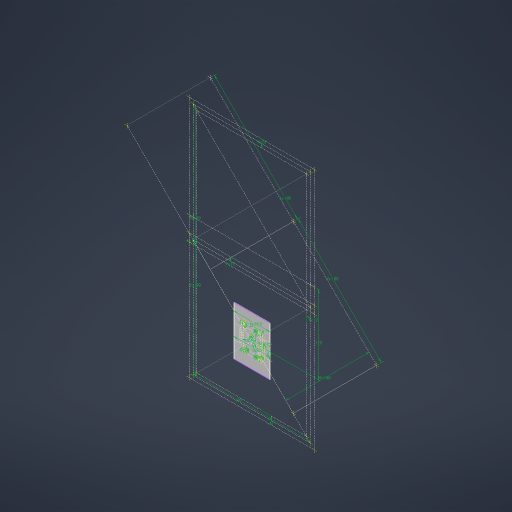
# Autodesk Inventor part: chassis
Saved by Autodesk Inventor 2023.5 (Build 275446000, 446)
## iProperties
Created: 2025-01-19
Part Number: chassis
Material: 一般
Document SubType Name: Modeling
Designer: IshiiLabHonda
Density: 1 g/cm^3
Appearance: 既定
Author: IshiiLabHonda
Autodesk Inventor part; units mm, degrees
ref_plane "YZ Plane" through (0, 0, 0) normal (1, 0, 0) x (0, 1, 0)
ref_plane "XZ Plane" through (0, 0, 0) normal (0, 1, 0) x (-1, 0, 0)
ref_plane "XY Plane" through (0, 0, 0) normal (0, 0, 1) x (1, 0, 0)
sketch "スケッチ1" plane through (0, 0, 0) normal (0, 0, 1) x (1, 0, 0)
  line L0 (-90, 90) -> (90, 90) construction
  line L1 (90, 90) -> (90, -90) construction
  line L2 (90, -90) -> (-90, -90) construction
  line L3 (-90, -90) -> (-90, 90) construction
  line L4 (-90, 90) -> (-90, 270) construction
  line L5 (-90, 270) -> (90, 270) construction
  line L6 (90, 270) -> (90, 90) construction
  line L7 (-90, 90) -> (90, -90) construction
  line L8 (90, 90) -> (-90, -90) construction
  line L9 (0, 0) -> (0, 10) construction
  line L10 (0, 0) -> (10, 0) construction
  line L11 (-90, 270) -> (90, 90) construction
  line L12 (-90, 90) -> (90, 270) construction
  line L13 (-96, 276) -> (96, 276) construction
  line L14 (96, 276) -> (96, -96) construction
  line L15 (96, -96) -> (-96, -96) construction
  line L16 (-96, -96) -> (-96, 276) construction
  line L17 (-84, 264) -> (84, 264) construction
  line L18 (84, 264) -> (84, -84) construction
  line L19 (84, -84) -> (-84, -84) construction
  line L20 (-84, -84) -> (-84, 264) construction
  line L21 (-96, 96) -> (96, 96) construction
  line L22 (-96, 84) -> (96, 84) construction
  line L23 (-63.6396, 63.6396) -> (63.6396, 190.9188) construction
  line L24 (63.6396, 190.9188) -> (190.9188, 63.6396) construction
  line L25 (190.9188, 63.6396) -> (63.6396, -63.6396) construction
  line L26 (63.6396, -63.6396) -> (-63.6396, 63.6396) construction
  line L27 (-190.9188, 190.9188) -> (-63.6396, 318.1981) construction
  line L28 (-63.6396, 318.1981) -> (63.6396, 190.9188) construction
  line L29 (-63.6396, 63.6396) -> (-190.9188, 190.9188) construction
  line L30 (-96, 120) -> (96, 120) construction
  point P0 (-63.6396, 318.1981)
  point P1 (-90, 120)
  point P2 (90, 120)
  dimension "d8" = 10
  dimension "d9" = 10
  dimension "d10" = 12
  dimension "d11" = 12
  dimension "d12" = 12
  dimension "d13" = 12
  dimension "d14" = 180
  dimension "d15" = 180
  dimension "d16" = 180
  dimension "d17" = 12
  dimension "d34" = 180
  dimension "d35" = 180
  dimension "d36" = 180
  dimension "d37" = 120
  constraints: 62 end point, 13 parallel, 10 point on line, 9 perpendicular, 3 coincident, 2 midpoint, 1 horizontal, 6 other
  measures "d8" distance of L9.start L9.end
  measures "d9" distance of L9.start L10.end
  measures "d10" distance between parallel lines of L15 L19
  measures "d11" distance between parallel lines of L16 L20
  measures "d12" distance between parallel lines of L14 L18
  measures "d13" distance between parallel lines of L17 L13
  measures "d14" distance of L1.end L2.end
  measures "d15" distance of L2.end L0.start
  measures "d16" distance between parallel lines of L0 L5
  measures "d17" distance between parallel lines of L22 L21
  measures "d34" distance between parallel lines of L26 L24
  measures "d35" distance of L23.end L24.end
  measures "d36" distance between parallel lines of L23 L27
  measures "d37" distance between parallel lines of L10 L30
sketch "スケッチ2" plane through (0, 0, 0) normal (0, 0, 1) x (1, 0, 0)
  line L0 (63.6396, 190.9188) -> (190.9188, 63.6396) construction
  line L1 (-63.6396, 318.1981) -> (63.6396, 190.9188) construction
  line L2 (-84, 264) -> (84, 264) construction
  line L3 (-90, 270) -> (90, 270) construction
  line L4 (90, 270) -> (90, 90) construction
  line L5 (-96, 276) -> (96, 276) construction
  line L6 (-90, 90) -> (90, 270) construction
  line L7 (-90, 270) -> (90, 90) construction
  line L8 (-63.6396, 63.6396) -> (63.6396, 190.9188) construction
  line L9 (-96, 120) -> (96, 120) construction
  line L10 (-90, 90) -> (90, 90) construction
  line L11 (-96, 96) -> (96, 96) construction
  line L12 (-96, 84) -> (96, 84) construction
  line L13 (90, -90) -> (-90, -90) construction
  line L14 (0, 0) -> (0, 10) construction
  line L15 (0, 0) -> (10, 0) construction
  line L16 (190.9188, 63.6396) -> (63.6396, -63.6396) construction
  line L17 (63.6396, -63.6396) -> (-63.6396, 63.6396) construction
  line L18 (84, -84) -> (-84, -84) construction
  line L19 (96, -96) -> (-96, -96) construction
  line L20 (-90, 90) -> (-90, 270) construction
  line L21 (-63.6396, 63.6396) -> (-190.9188, 190.9188) construction
  line L22 (-190.9188, 190.9188) -> (-63.6396, 318.1981) construction
  line L23 (96, 276) -> (96, -96) construction
  line L24 (-96, -96) -> (-96, 276) construction
  line L25 (84, 264) -> (84, -84) construction
  line L26 (-84, -84) -> (-84, 264) construction
  line L27 (90, 90) -> (90, -90) construction
  line L28 (-90, 90) -> (90, -90) construction
  line L29 (90, 90) -> (-90, -90) construction
  line L30 (-90, -90) -> (-90, 90) construction
  circle A0 centre (0, 0) radius 15 construction
  circle A1 centre (0, 0) radius 7.5 construction
  line L31 (19, 11.5) -> (27.75, 11.5) construction
  line L32 (27.75, 11.5) -> (27.75, -11.5) construction
  line L33 (27.75, -11.5) -> (19, -11.5) construction
  line L34 (19, -11.5) -> (19, 11.5) construction
  line L35 (19, 11.5) -> (17, 11.5) construction
  line L36 (17, 11.5) -> (17, -11.5) construction
  line L37 (17, -11.5) -> (19, -11.5) construction
  line L38 (17, 1.5) -> (16, 1.5) construction
  line L39 (16, -1.5) -> (17, -1.5) construction
  line L40 (-16, 20) -> (16, 20) construction
  line L41 (16, 20) -> (16, -20) construction
  line L42 (16, -20) -> (-16, -20) construction
  line L43 (-16, -20) -> (-16, 20) construction
  line L44 (-19, 11.5) -> (-27.75, 11.5) construction
  line L45 (-27.75, 11.5) -> (-27.75, -11.5) construction
  line L46 (-27.75, -11.5) -> (-19, -11.5) construction
  line L47 (-19, -11.5) -> (-19, 11.5) construction
  line L48 (-19, 11.5) -> (-17, 11.5) construction
  line L49 (-17, 11.5) -> (-17, -11.5) construction
  line L50 (-17, -11.5) -> (-19, -11.5) construction
  line L51 (-17, 1.5) -> (-16, 1.5) construction
  line L52 (-16, -1.5) -> (-17, -1.5) construction
  line L53 (-13.5, 20) -> (-13.5, -20) construction
  line L54 (13.5, 20) -> (13.5, -20) construction
  line L55 (-9.5, 20) -> (-9.5, 15) construction
  line L56 (-9.5, 15) -> (-13.5, 15) construction
  line L57 (-13.5, 20) -> (-9.5, 15) construction
  line L58 (-9.5, 20) -> (-13.5, 15) construction
  circle A2 centre (-11.5, 17.5) radius 0.8 construction
  line L59 (9.5, 20) -> (9.5, 15) construction
  line L60 (9.5, 15) -> (13.5, 15) construction
  line L61 (9.5, 20) -> (13.5, 15) construction
  line L62 (9.5, 15) -> (13.5, 20) construction
  circle A3 centre (11.5, 17.5) radius 0.8 construction
  line L63 (-13.5, -15) -> (-9.5, -15) construction
  line L64 (-9.5, -15) -> (-9.5, -20) construction
  line L65 (9.5, -20) -> (9.5, -15) construction
  line L66 (9.5, -15) -> (13.5, -15) construction
  line L67 (-13.5, -15) -> (-9.5, -20) construction
  line L68 (-9.5, -15) -> (-13.5, -20) construction
  circle A4 centre (-11.5, -17.5) radius 0.8 construction
  line L69 (9.5, -15) -> (13.5, -20) construction
  line L70 (13.5, -15) -> (9.5, -20) construction
  circle A5 centre (11.5, -17.5) radius 0.8 construction
  point P0 (90, 120)
  point P1 (-90, 120)
  point P2 (-63.6396, 318.1981)
  dimension "d38" = 30
  dimension "d39" = 15
  dimension "d40" = 8.75
  dimension "d41" = 2
  dimension "d42" = 23
  dimension "d44" = 3
  dimension "d45" = 1
  dimension "d46" = 32
  dimension "d48" = 2.5
  dimension "d49" = 20
  dimension "d50" = 20
  dimension "d51" = 1.6
  dimension "d52" = 5
  dimension "d53" = 4
  dimension "d54" = 1.6
  dimension "d55" = 4
  dimension "d56" = 5
  dimension "d57" = 1.6
  dimension "d58" = 4
  dimension "d59" = 5
  dimension "d60" = 1.6
  dimension "d61" = 5
  dimension "d62" = 4
  dimension "d63" = 55.5
  constraints: 80 end point, 18 point on line, 12 parallel, 10 symmetric about line, 6 centre point, 6 perpendicular, 4 midpoint, 2 coincident, 2 collinear, 5 other
  measures "d38" diameter of A0
  measures "d39" diameter of A1
  measures "d40" distance between parallel lines of L34 L32
  measures "d41" distance between parallel lines of L36 L34
  measures "d42" distance between parallel lines of L33 L31
  measures "d44" distance between parallel lines of L39 L38
  measures "d45" distance between parallel lines of L41 L36
  measures "d46" distance between parallel lines of L41 L43
  measures "d48" distance between parallel lines of L43 L53
  measures "d49" distance between parallel lines of L42 L15
  measures "d50" distance between parallel lines of L15 L40
  measures "d51" diameter of A2
  measures "d52" distance of L55.start L55.end
  measures "d53" distance of L55.end L56.end
  measures "d54" diameter of A3
  measures "d55" distance of L59.end L60.end
  measures "d56" distance of L59.start L59.end
  measures "d57" diameter of A4
  measures "d58" distance of L63.start L63.end
  measures "d59" distance of L63.end L64.end
  measures "d60" diameter of A5
  measures "d61" distance of L65.start L65.end
  measures "d62" distance of L65.end L66.end
  measures "d63" distance between parallel lines of L32 L45
sketch "スケッチ3" plane through (0, 0, 0) normal (0, 0, 1) x (1, 0, 0)
  line L0 (63.6396, 190.9188) -> (190.9188, 63.6396) construction
  line L1 (-63.6396, 318.1981) -> (63.6396, 190.9188) construction
  line L2 (-84, 264) -> (84, 264) construction
  line L3 (-90, 270) -> (90, 270) construction
  line L4 (90, 270) -> (90, 90) construction
  line L5 (-96, 276) -> (96, 276) construction
  line L6 (-90, 90) -> (90, 270) construction
  line L7 (-90, 270) -> (90, 90) construction
  line L8 (-63.6396, 63.6396) -> (63.6396, 190.9188) construction
  line L9 (-96, 120) -> (96, 120) construction
  line L10 (-90, 90) -> (90, 90) construction
  line L11 (-96, 96) -> (96, 96) construction
  line L12 (-96, 84) -> (96, 84) construction
  line L13 (90, -90) -> (-90, -90) construction
  line L14 (0, 0) -> (0, 10) construction
  line L15 (0, 0) -> (10, 0) construction
  line L16 (190.9188, 63.6396) -> (63.6396, -63.6396) construction
  line L17 (63.6396, -63.6396) -> (-63.6396, 63.6396) construction
  line L18 (84, -84) -> (-84, -84) construction
  line L19 (96, -96) -> (-96, -96) construction
  line L20 (-90, 90) -> (-90, 270) construction
  line L21 (-63.6396, 63.6396) -> (-190.9188, 190.9188) construction
  line L22 (-190.9188, 190.9188) -> (-63.6396, 318.1981) construction
  line L23 (96, 276) -> (96, -96) construction
  line L24 (-96, -96) -> (-96, 276) construction
  line L25 (84, 264) -> (84, -84) construction
  line L26 (-84, -84) -> (-84, 264) construction
  line L27 (90, 90) -> (90, -90) construction
  line L28 (-90, 90) -> (90, -90) construction
  line L29 (90, 90) -> (-90, -90) construction
  line L30 (-90, -90) -> (-90, 90) construction
  line L31 (-17, 1.5) -> (-16, 1.5) construction
  line L32 (-16, -1.5) -> (-17, -1.5) construction
  line L33 (-19, 11.5) -> (-17, 11.5) construction
  line L34 (-27.75, 11.5) -> (-27.75, -11.5) construction
  line L35 (63.6396, -63.6396) -> (-63.6396, 63.6396) construction
  line L36 (84, -84) -> (-84, -84) construction
  line L37 (-90, -90) -> (-90, 90) construction
  line L38 (96, -96) -> (-96, -96) construction
  line L39 (-90, 90) -> (90, 90) construction
  line L40 (90, -90) -> (-90, -90) construction
  line L41 (90, 90) -> (-90, -90) construction
  line L42 (-90, 90) -> (90, -90) construction
  line L43 (90, 90) -> (90, -90) construction
  line L44 (-27.75, -11.5) -> (-19, -11.5) construction
  line L45 (-19, 11.5) -> (-27.75, 11.5) construction
  line L46 (-17, 11.5) -> (-17, -11.5) construction
  line L47 (-17, -11.5) -> (-19, -11.5) construction
  line L48 (0, 0) -> (0, 10) construction
  line L49 (0, 0) -> (10, 0) construction
  circle A0 centre (0, 0) radius 15 construction
  circle A1 centre (0, 0) radius 7.5 construction
  line L50 (-13.5, 20) -> (-13.5, -20) construction
  line L51 (-16, 20) -> (16, 20) construction
  line L52 (-16, -20) -> (-16, 20) construction
  line L53 (16, -20) -> (-16, -20) construction
  line L54 (-13.5, -15) -> (-9.5, -15) construction
  circle A2 centre (-11.5, -17.5) radius 0.8 projected
  line L55 (-9.5, -15) -> (-13.5, -20) construction
  line L56 (-13.5, -15) -> (-9.5, -20) construction
  line L57 (-63.6396, 318.1981) -> (63.6396, 190.9188) construction
  line L58 (-84, 264) -> (84, 264) construction
  line L59 (-90, 270) -> (90, 270) construction
  line L60 (90, 270) -> (90, 90) construction
  line L61 (-96, 276) -> (96, 276) construction
  line L62 (-90, 90) -> (90, 270) construction
  line L63 (-90, 270) -> (90, 90) construction
  line L64 (-63.6396, 63.6396) -> (63.6396, 190.9188) construction
  line L65 (-96, 120) -> (96, 120) construction
  line L66 (-96, 96) -> (96, 96) construction
  line L67 (-96, 84) -> (96, 84) construction
  line L68 (84, 264) -> (84, -84) construction
  line L69 (96, 276) -> (96, -96) construction
  line L70 (-96, -96) -> (-96, 276) construction
  line L71 (-84, -84) -> (-84, 264) construction
  line L72 (-63.6396, 63.6396) -> (-190.9188, 190.9188) construction
  line L73 (-90, 90) -> (-90, 270) construction
  line L74 (-190.9188, 190.9188) -> (-63.6396, 318.1981) construction
  line L75 (-19, -11.5) -> (-19, 11.5) construction
  line L76 (9.5, -15) -> (13.5, -15) construction
  line L77 (9.5, -20) -> (9.5, -15) construction
  circle A3 centre (11.5, -17.5) radius 0.8 projected
  line L78 (9.5, -15) -> (13.5, -20) construction
  line L79 (13.5, -15) -> (9.5, -20) construction
  line L80 (-9.5, -15) -> (-9.5, -20) construction
  line L81 (63.6396, 190.9188) -> (190.9188, 63.6396) construction
  line L82 (190.9188, 63.6396) -> (63.6396, -63.6396) construction
  line L83 (19, 11.5) -> (27.75, 11.5) construction
  line L84 (27.75, 11.5) -> (27.75, -11.5) construction
  line L85 (16, -1.5) -> (17, -1.5) construction
  line L86 (17, -11.5) -> (19, -11.5) construction
  line L87 (27.75, -11.5) -> (19, -11.5) construction
  line L88 (13.5, 20) -> (13.5, -20) construction
  line L89 (16, 20) -> (16, -20) construction
  line L90 (17, 11.5) -> (17, -11.5) construction
  line L91 (19, -11.5) -> (19, 11.5) construction
  line L92 (19, 11.5) -> (17, 11.5) construction
  line L93 (17, 1.5) -> (16, 1.5) construction
  line L94 (-9.5, 20) -> (-9.5, 15) construction
  line L95 (9.5, 15) -> (13.5, 15) construction
  circle A4 centre (11.5, 17.5) radius 0.8 projected
  line L96 (9.5, 20) -> (13.5, 15) construction
  line L97 (9.5, 15) -> (13.5, 20) construction
  line L98 (9.5, 20) -> (9.5, 15) construction
  line L99 (-9.5, 15) -> (-13.5, 15) construction
  circle A5 centre (-11.5, 17.5) radius 0.8 projected
  line L100 (-13.5, 20) -> (-9.5, 15) construction
  line L101 (-9.5, 20) -> (-13.5, 15) construction
  line L102 (-27.75, 38.248) -> (27.75, 38.248)
  line L103 (27.75, 38.248) -> (27.75, -36.8074)
  line L104 (27.75, -36.8074) -> (-27.75, -36.8074)
  line L105 (-27.75, -36.8074) -> (-27.75, 38.248)
  point P0 (90, 120)
  point P1 (-90, 120)
  point P2 (-63.6396, 318.1981)
  point P3 (-63.6396, 318.1981)
  point P4 (-90, 120)
  point P5 (90, 120)
  dimension "d64" = 55.5
  constraints: 8 end point, 3 parallel, 1 perpendicular, 14 other
  measures "d64" distance between parallel lines of L103 L105
extrude "押し出し1" add sketch "スケッチ3" against normal blind 1 contours A2 | A3 | A4 | A5 | L102 L103 L104 L105
extrude "押し出し2" cut sketch "スケッチ3" against normal blind 1 contours A2 | A3 | A4 | A5
equation "\"d9\" = d8"
equation "\"d11\" = d10"
equation "\"d12\" = d10"
equation "\"d13\" = d10"
equation "\"d15\" = d14"
equation "\"d16\" = d14"
equation "\"d17\" = d10"
